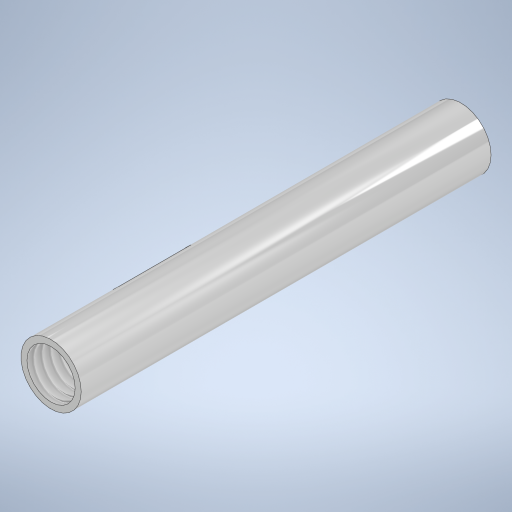
# Autodesk Inventor part: shaft_34mm_Φ5
Saved by Autodesk Inventor 2024 (Build 280153000, 153)
## iProperties
Created: 2025-06-13
Part Number: shaft_34mm_Φ5
Material: アルミニウム 7075
Document SubType Name: Modeling
Designer: 1412z
Density: 2.81 g/cm^3
Appearance: アルミニウム - つや出し
Author: 1412z
Autodesk Inventor part; units mm, degrees
ref_plane "YZ Plane" through (0, 0, 0) normal (1, 0, 0) x (0, 1, 0)
ref_plane "XZ Plane" through (0, 0, 0) normal (0, 1, 0) x (-1, 0, 0)
ref_plane "XY Plane" through (0, 0, 0) normal (0, 0, 1) x (1, 0, 0)
sketch "スケッチ1" plane through (0, 0, 0) normal (0, 0, 1) x (1, 0, 0)
  circle A0 centre (0, 0) radius 2.5
  dimension "d0" = 5
  constraints: 1 centre point, 1 coincident
  measures "d0" diameter of A0
extrude "押し出し1" add sketch "スケッチ1" along normal blind 34
sketch "スケッチ2" plane through (0, 0, 34) normal (0, 0, 1) x (1, 0, 0)
  circle A0 centre (0, 0) radius 2
  dimension "d3" = 4
  constraints: 1 centre point, 1 coincident
  measures "d3" diameter of A0
extrude "押し出し2" cut sketch "スケッチ2" against normal blind 6
thread "ねじ1" size "M4x0.7" class "6H" standard "ANSI Metric M Profile" full length
sketch "スケッチ3" plane through (0, 0, 0) normal (0, 1, 0) x (-1, 0, 0)
  line L0 (2.5, 0) -> (2.5, 34) projected
  line L1 (2.5, 23.9) -> (2.5, 26.9)
  line L2 (2.5, 26.9) -> (1.5, 26.9)
  line L3 (1.5, 26.9) -> (1.5, 20.9)
  line L4 (1.5, 20.9) -> (2.5, 20.9)
  line L5 (2.5, 20.9) -> (2.5, 23.9)
  point P0 (0, 0)
  dimension "d8" = 3
  dimension "d9" = 1
  dimension "d10" = 6
  constraints: 10 end point, 4 perpendicular, 2 point on line, 1 vertical
  measures "d8" distance of L1.start L1.end
  measures "d9" distance of L1.end L2.end
  measures "d10" distance of L2.end L3.end
extrude "押し出し3" cut sketch "スケッチ3" along normal mid plane 10
